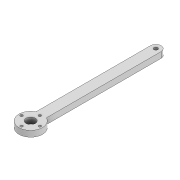
# Autodesk Inventor part: Wing_arm_1
Saved by Autodesk Inventor 2022 (Build 260153000, 153)
## iProperties
Created: 2022-07-06
Part Number: Wing_arm_1
Material: Generic
Document SubType Name: Modeling
Designer: dell
Density: 1 g/cm^3
Appearance: Default
Author: dell
Autodesk Inventor part; units mm, degrees
ref_plane "YZ Plane" through (0, 0, 0) normal (1, 0, 0) x (0, 1, 0)
ref_plane "XZ Plane" through (0, 0, 0) normal (0, 1, 0) x (-1, 0, 0)
ref_plane "XY Plane" through (0, 0, 0) normal (0, 0, 1) x (1, 0, 0)
sketch "Sketch1" plane through (0, 0, 0) normal (0, 1, 0) x (-1, 0, 0)
  circle A0 centre (0, 0) radius 9
  circle A1 centre (0, 0) radius 3.55
  circle A2 centre (7, 0) radius 1
  circle A3 centre (0, 7) radius 1
  circle A4 centre (-7, 0) radius 1
  circle A5 centre (0, -7) radius 1
  dimension "d0" = 18
  dimension "d1" = 7.1
  dimension "d2" = 2
  dimension "d3" = 7
  dimension "d6" = 360
  constraints: 6 centre point, 2 coincident, 9 other
  measures "d0" diameter of A0
  measures "d1" diameter of A1
  measures "d2" diameter of A2
  measures "d3" distance of point (0, 0) A2.centre
extrude "Extrusion1" add sketch "Sketch1" along normal blind 4.5
sketch "Sketch4" plane through (0, 0, 0) normal (0, -1, 0) x (1, 0, 0)
  line L0 (0, 0) -> (0, -95.811) construction
  line L1 (-4, 0) -> (-4, -95.811)
  line L2 (4, -95.811) -> (4, 0)
  arc A0 (4, 0) -> (-4, 0) centre (0, 0) ccw
  arc A1 (-4, -95.811) -> (4, -95.811) centre (0, -95.811) ccw
  circle A2 centre (0, -95.811) radius 1.5
  circle A3 centre (0, 0) radius 9 projected
  circle A4 centre (0, -7) radius 1 projected
  circle A5 centre (7, 0) radius 1 projected
  circle A6 centre (0, 7) radius 1 projected
  circle A7 centre (-7, 0) radius 1 projected
  circle A8 centre (0, 0) radius 3.55 projected
  point P0 (0, -47.9055)
  point P1 (4, -8.0623)
  point P2 (-4, -8.0623)
  dimension "d19" = 95.811
  dimension "d20" = 8
  dimension "d21" = 3
  constraints: 8 end point, 4 point on circle, 4 tangent, 3 centre point, 1 coincident, 1 midpoint, 1 parallel, 1 vertical
  measures "d19" distance of L0.start L0.end
  measures "d20" diameter of A1
  measures "d21" diameter of A2
extrude "Extrusion4" add sketch "Sketch4" against normal blind 4.5 contours A3 L2 A1 L1
body "Solid1"
